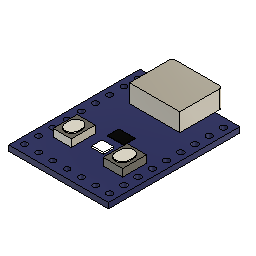
Waveshare RP2040 Zero (Autodesk Fusion 360 design; units mm, degrees)
Autodesk Fusion 360 part; units mm, degrees
sketch "Sketch1" plane through (0, 0, 0) normal (0, 0, 1) x (1, 0, 0)
  line L0 (-8.481, 10.9754) -> (9.5262, 10.9754)
  line L1 (9.5262, 10.9754) -> (9.5262, -12.7333)
  line L2 (9.5262, -12.7333) -> (-8.481, -12.7333)
  line L3 (-8.481, -12.7333) -> (-8.481, 10.9754)
  constraint horizontal L0
  constraint vertical L1
  constraint horizontal L2
  constraint vertical L3
extrude "Extrude1" add sketch "Sketch1" along normal blind 1
sketch "Sketch2" plane through (0, 0, 1) normal (0, 0, 1) x (-1, 0, 0)
  line L0 (8.481, 12.7333) -> (-9.5262, 12.7333)
  line L1 (-9.5262, 12.7333) -> (-9.5262, -10.9754)
  line L2 (-9.5262, -10.9754) -> (8.481, -10.9754)
  line L3 (8.481, -10.9754) -> (8.481, 12.7333)
  line L4 (4.0143, -12.313) -> (-5.0507, -12.313)
  line L5 (-5.0507, -12.313) -> (-5.0507, -4.6154)
  line L6 (-5.0507, -4.6154) -> (4.0143, -4.6154)
  line L7 (4.0143, -4.6154) -> (4.0143, -12.313)
  dimension "d3" = 9.065
  constraint horizontal L4
  constraint vertical L5
  constraint horizontal L6
  constraint vertical L7
  measures "d3" distance of L4.start L4.end
extrude "Extrude2" add sketch "Sketch2" along normal blind 3.27 contours L2 L4 L5 L7 | L2 L5 L6 L7
sketch "Sketch3" plane through (0, 0, 1) normal (0, 0, 1) x (-1, 0, 0)
  line L0 (4.0143, -4.6154) -> (4.0143, -10.9754)
  line L1 (4.0143, -10.9754) -> (8.481, -10.9754)
  line L2 (8.481, -10.9754) -> (8.481, 12.7333)
  line L3 (8.481, 12.7333) -> (-9.5262, 12.7333)
  line L4 (-9.5262, 12.7333) -> (-9.5262, -10.9754)
  line L5 (-9.5262, -10.9754) -> (-5.0507, -10.9754)
  line L6 (-5.0507, -10.9754) -> (-5.0507, -4.6154)
  line L7 (-5.0507, -4.6154) -> (4.0143, -4.6154)
  circle A0 centre (7.1853, -9.3478) radius 0.5131
  circle A1 centre (7.1853, -6.7791) radius 0.5131
  circle A2 centre (7.1853, -4.2103) radius 0.5131
  circle A3 centre (7.1853, -1.6416) radius 0.5131
  circle A4 centre (7.1853, 0.9272) radius 0.5131
  circle A5 centre (7.1853, 3.4959) radius 0.5131
  circle A6 centre (7.1853, 6.0647) radius 0.5131
  circle A7 centre (7.1853, 8.6334) radius 0.5131
  circle A8 centre (7.1853, 11.2022) radius 0.5131
  dimension "d8" = 0
  dimension "d9" = 20.55
extrude "Extrude3" cut sketch "Sketch3" against normal blind 1 contours A0 | A1 | A2 | A3 | A4 | A5 | A6 | A7 | A8
sketch "Sketch4" plane through (0, 12.313, 0) normal (0, 1, 0) x (-1, 0, 0)
  line L0 (-5.0507, 1) -> (4.0143, 1)
  line L1 (4.0143, 1) -> (4.0143, 4.27)
  line L2 (4.0143, 4.27) -> (-5.0507, 4.27)
  line L3 (-5.0507, 4.27) -> (-5.0507, 1)
  line L4 (-4.7493, 3.8918) -> (3.7026, 3.8918)
  line L5 (3.7026, 3.8918) -> (3.7026, 1.2313)
  line L6 (3.7026, 1.2313) -> (-4.7493, 1.2313)
  line L7 (-4.7493, 1.2313) -> (-4.7493, 3.8918)
  dimension "d12" = 8.4519
  constraint horizontal L4
  constraint vertical L5
  constraint horizontal L6
  constraint vertical L7
  measures "d12" distance of L4.start L4.end
extrude "Extrude4" cut sketch "Sketch4" against normal blind 7 contours L4 L5 L6 L7
sketch "Sketch5" plane through (0, 5.313, 0) normal (0, 1, 0) x (-1, 0, 0)
  line L0 (-4.7493, 1.2313) -> (3.7026, 1.2313)
  line L1 (3.7026, 1.2313) -> (3.7026, 3.8918)
  line L2 (3.7026, 3.8918) -> (-4.7493, 3.8918)
  line L3 (-4.7493, 3.8918) -> (-4.7493, 1.2313)
  line L4 (-4.1571, 2.6965) -> (3.1998, 2.6965)
  line L5 (3.1998, 2.6965) -> (3.1998, 2.1768)
  line L6 (3.1998, 2.1768) -> (-4.1571, 2.1768)
  line L7 (-4.1571, 2.1768) -> (-4.1571, 2.6965)
  constraint horizontal L4
  constraint vertical L5
  constraint horizontal L6
  constraint vertical L7
extrude "Extrude5" add sketch "Sketch5" along normal blind 7 contours L4 L5 L6 L7
fillet "Fillet1" radius 0.45 1 edges at (5.0507, 12.313, 2.635)
fillet "Fillet2" radius 0.7 1 edges at (-4.0143, 12.313, 2.635)
sketch "Sketch6" plane through (0, 0, 1) normal (0, 0, 1) x (-1, 0, 0)
  circle A0 centre (7.1853, -4.2103) radius 0.5131
  circle A1 centre (7.1853, 6.0647) radius 0.5131
  circle A2 centre (7.1853, 8.6334) radius 0.5131
  circle A3 centre (7.1853, -1.6416) radius 0.5131
  circle A4 centre (7.1853, -6.7791) radius 0.5131
  circle A5 centre (7.1853, 3.4959) radius 0.5131
  circle A6 centre (7.1853, 11.2022) radius 0.5131
  circle A7 centre (7.1853, 0.9272) radius 0.5131
  circle A8 centre (7.1853, -9.3478) radius 0.5131
  line L0 (4.0143, -4.6154) -> (4.0143, -10.9754)
  line L1 (4.0143, -10.9754) -> (8.481, -10.9754)
  line L2 (8.481, -10.9754) -> (8.481, 12.7333)
  line L3 (8.481, 12.7333) -> (-9.5262, 12.7333)
  line L4 (-9.5262, 12.7333) -> (-9.5262, -10.9754)
  line L5 (-9.5262, -10.9754) -> (-5.0507, -10.9754)
  line L6 (-5.0507, -10.9754) -> (-5.0507, -4.6154)
  line L7 (-5.0507, -4.6154) -> (4.0143, -4.6154)
  circle A9 centre (-8.1988, -9.3488) radius 0.5473
  circle A10 centre (-8.1988, -6.78) radius 0.5473
  circle A11 centre (-8.1988, -4.2113) radius 0.5473
  circle A12 centre (-8.1988, -1.6425) radius 0.5473
  circle A13 centre (-8.1988, 0.9262) radius 0.5473
  circle A14 centre (-8.1988, 3.495) radius 0.5473
  circle A15 centre (-8.1988, 6.0637) radius 0.5473
  circle A16 centre (-8.1988, 8.6325) radius 0.5473
  circle A17 centre (-8.1988, 11.2012) radius 0.5473
  dimension "d23" = 0
  dimension "d24" = 20.55
extrude "Extrude6" cut sketch "Sketch6" against normal blind 1 contours A9 | A10 | A11 | A12 | A13 | A14 | A15 | A16 | A17
sketch "Sketch7" plane through (0, 0, 1) normal (0, 0, 1) x (-1, 0, 0)
  circle A0 centre (-8.1988, 6.0637) radius 0.5473
  circle A1 centre (-8.1988, -4.2113) radius 0.5473
  circle A2 centre (-8.1988, -6.78) radius 0.5473
  circle A3 centre (-8.1988, 3.495) radius 0.5473
  circle A4 centre (-8.1988, 8.6325) radius 0.5473
  circle A5 centre (-8.1988, -1.6425) radius 0.5473
  circle A6 centre (-8.1988, -9.3488) radius 0.5473
  circle A7 centre (-8.1988, 0.9262) radius 0.5473
  circle A8 centre (-8.1988, 11.2012) radius 0.5473
  circle A9 centre (7.1853, -4.2103) radius 0.5131
  circle A10 centre (7.1853, 6.0647) radius 0.5131
  circle A11 centre (7.1853, 8.6334) radius 0.5131
  circle A12 centre (7.1853, -1.6416) radius 0.5131
  circle A13 centre (7.1853, -6.7791) radius 0.5131
  circle A14 centre (7.1853, 3.4959) radius 0.5131
  circle A15 centre (7.1853, 11.2022) radius 0.5131
  circle A16 centre (7.1853, 0.9272) radius 0.5131
  circle A17 centre (7.1853, -9.3478) radius 0.5131
  line L0 (4.0143, -4.6154) -> (4.0143, -10.9754)
  line L1 (4.0143, -10.9754) -> (8.481, -10.9754)
  line L2 (8.481, -10.9754) -> (8.481, 12.7333)
  line L3 (8.481, 12.7333) -> (-9.5262, 12.7333)
  line L4 (-9.5262, 12.7333) -> (-9.5262, -10.9754)
  line L5 (-9.5262, -10.9754) -> (-5.0507, -10.9754)
  line L6 (-5.0507, -10.9754) -> (-5.0507, -4.6154)
  line L7 (-5.0507, -4.6154) -> (4.0143, -4.6154)
  circle A18 centre (-5.6867, 11.2133) radius 0.5016
  circle A19 centre (-3.1117, 11.2133) radius 0.5016
  circle A20 centre (-0.5367, 11.2133) radius 0.5016
  circle A21 centre (2.0383, 11.2133) radius 0.5016
  circle A22 centre (4.6133, 11.2133) radius 0.5016
  dimension "d27" = 1.0031
  dimension "d30" = 10.3
  dimension "d31" = 0
  measures "d27" diameter of A18
extrude "Extrude7" cut sketch "Sketch7" against normal blind 1 contours A18 | A19 | A20 | A21 | A22
sketch "Sketch8" plane through (0, 0, 1) normal (0, 0, 1) x (-1, 0, 0)
  circle A0 centre (-0.5367, 11.2133) radius 0.5016
  circle A1 centre (2.0383, 11.2133) radius 0.5016
  circle A2 centre (-3.1117, 11.2133) radius 0.5016
  circle A3 centre (4.6133, 11.2133) radius 0.5016
  circle A4 centre (-5.6867, 11.2133) radius 0.5016
  circle A5 centre (-8.1988, 6.0637) radius 0.5473
  circle A6 centre (-8.1988, -4.2113) radius 0.5473
  circle A7 centre (-8.1988, -6.78) radius 0.5473
  circle A8 centre (-8.1988, 3.495) radius 0.5473
  circle A9 centre (-8.1988, 8.6325) radius 0.5473
  circle A10 centre (-8.1988, -1.6425) radius 0.5473
  circle A11 centre (-8.1988, -9.3488) radius 0.5473
  circle A12 centre (-8.1988, 0.9262) radius 0.5473
  circle A13 centre (-8.1988, 11.2012) radius 0.5473
  circle A14 centre (7.1853, -4.2103) radius 0.5131
  circle A15 centre (7.1853, 6.0647) radius 0.5131
  circle A16 centre (7.1853, 8.6334) radius 0.5131
  circle A17 centre (7.1853, -1.6416) radius 0.5131
  circle A18 centre (7.1853, -6.7791) radius 0.5131
  circle A19 centre (7.1853, 3.4959) radius 0.5131
  circle A20 centre (7.1853, 11.2022) radius 0.5131
  circle A21 centre (7.1853, 0.9272) radius 0.5131
  circle A22 centre (7.1853, -9.3478) radius 0.5131
  line L0 (4.0143, -4.6154) -> (4.0143, -10.9754)
  line L1 (4.0143, -10.9754) -> (8.481, -10.9754)
  line L2 (8.481, -10.9754) -> (8.481, 12.7333)
  line L3 (8.481, 12.7333) -> (-9.5262, 12.7333)
  line L4 (-9.5262, 12.7333) -> (-9.5262, -10.9754)
  line L5 (-9.5262, -10.9754) -> (-5.0507, -10.9754)
  line L6 (-5.0507, -10.9754) -> (-5.0507, -4.6154)
  line L7 (-5.0507, -4.6154) -> (4.0143, -4.6154)
  line L8 (2.4326, 7.493) -> (5.7199, 7.493)
  line L9 (5.7199, 7.493) -> (5.7199, 3.1598)
  line L10 (5.7199, 3.1598) -> (2.4326, 3.1598)
  line L11 (2.4326, 3.1598) -> (2.4326, 7.493)
  line L12 (-6.8316, 7.493) -> (-3.3202, 7.493)
  line L13 (-3.3202, 7.493) -> (-3.3202, 3.1748)
  line L14 (-3.3202, 3.1748) -> (-6.8316, 3.1748)
  line L15 (-6.8316, 3.1748) -> (-6.8316, 7.493)
  constraint horizontal L8
  constraint vertical L9
  constraint horizontal L10
  constraint vertical L11
  constraint horizontal L12
  constraint vertical L13
  constraint horizontal L14
  constraint vertical L15
extrude "Extrude8" add sketch "Sketch8" along normal blind 1.34 contours L8 L9 L10 L11 | L12 L13 L14 L15
sketch "Sketch9" plane through (0, 0, 1) normal (0, 0, 1) x (-1, 0, 0)
  line L0 (-6.8316, 3.1748) -> (-6.8316, 7.493)
  line L1 (-6.8316, 7.493) -> (-3.3202, 7.493)
  line L2 (-3.3202, 7.493) -> (-3.3202, 3.1748)
  line L3 (-3.3202, 3.1748) -> (-6.8316, 3.1748)
  line L4 (2.4326, 3.1598) -> (2.4326, 7.493)
  line L5 (2.4326, 7.493) -> (5.7199, 7.493)
  line L6 (5.7199, 7.493) -> (5.7199, 3.1598)
  line L7 (5.7199, 3.1598) -> (2.4326, 3.1598)
  circle A0 centre (-0.5367, 11.2133) radius 0.5016
  circle A1 centre (2.0383, 11.2133) radius 0.5016
  circle A2 centre (-3.1117, 11.2133) radius 0.5016
  circle A3 centre (4.6133, 11.2133) radius 0.5016
  circle A4 centre (-5.6867, 11.2133) radius 0.5016
  circle A5 centre (-8.1988, 6.0637) radius 0.5473
  circle A6 centre (-8.1988, -4.2113) radius 0.5473
  circle A7 centre (-8.1988, -6.78) radius 0.5473
  circle A8 centre (-8.1988, 3.495) radius 0.5473
  circle A9 centre (-8.1988, 8.6325) radius 0.5473
  circle A10 centre (-8.1988, -1.6425) radius 0.5473
  circle A11 centre (-8.1988, -9.3488) radius 0.5473
  circle A12 centre (-8.1988, 0.9262) radius 0.5473
  circle A13 centre (-8.1988, 11.2012) radius 0.5473
  circle A14 centre (7.1853, -4.2103) radius 0.5131
  circle A15 centre (7.1853, 6.0647) radius 0.5131
  circle A16 centre (7.1853, 8.6334) radius 0.5131
  circle A17 centre (7.1853, -1.6416) radius 0.5131
  circle A18 centre (7.1853, -6.7791) radius 0.5131
  circle A19 centre (7.1853, 3.4959) radius 0.5131
  circle A20 centre (7.1853, 11.2022) radius 0.5131
  circle A21 centre (7.1853, 0.9272) radius 0.5131
  circle A22 centre (7.1853, -9.3478) radius 0.5131
  line L8 (4.0143, -4.6154) -> (4.0143, -10.9754)
  line L9 (4.0143, -10.9754) -> (8.481, -10.9754)
  line L10 (8.481, -10.9754) -> (8.481, 12.7333)
  line L11 (8.481, 12.7333) -> (-9.5262, 12.7333)
  line L12 (-9.5262, 12.7333) -> (-9.5262, -10.9754)
  line L13 (-9.5262, -10.9754) -> (-5.0507, -10.9754)
  line L14 (-5.0507, -10.9754) -> (-5.0507, -4.6154)
  line L15 (-5.0507, -4.6154) -> (4.0143, -4.6154)
  line L16 (-1.9669, 2.4371) -> (0.9625, 2.4371)
  line L17 (0.9625, 2.4371) -> (0.9625, 0.3676)
  line L18 (0.9625, 0.3676) -> (-1.9669, 0.3676)
  line L19 (-1.9669, 0.3676) -> (-1.9669, 2.4371)
  constraint horizontal L16
  constraint vertical L17
  constraint horizontal L18
  constraint vertical L19
extrude "Extrude9" add sketch "Sketch9" along normal blind 0.1 contours L16 L17 L18 L19
sketch "Sketch10" plane through (0, 0, 1) normal (0, 0, 1) x (-1, 0, 0)
  line L0 (-1.9669, 0.3676) -> (-1.9669, 2.4371)
  line L1 (-1.9669, 2.4371) -> (0.9625, 2.4371)
  line L2 (0.9625, 2.4371) -> (0.9625, 0.3676)
  line L3 (0.9625, 0.3676) -> (-1.9669, 0.3676)
  line L4 (-6.8316, 3.1748) -> (-6.8316, 7.493)
  line L5 (-6.8316, 7.493) -> (-3.3202, 7.493)
  line L6 (-3.3202, 7.493) -> (-3.3202, 3.1748)
  line L7 (-3.3202, 3.1748) -> (-6.8316, 3.1748)
  line L8 (2.4326, 3.1598) -> (2.4326, 7.493)
  line L9 (2.4326, 7.493) -> (5.7199, 7.493)
  line L10 (5.7199, 7.493) -> (5.7199, 3.1598)
  line L11 (5.7199, 3.1598) -> (2.4326, 3.1598)
  circle A0 centre (-0.5367, 11.2133) radius 0.5016
  circle A1 centre (2.0383, 11.2133) radius 0.5016
  circle A2 centre (-3.1117, 11.2133) radius 0.5016
  circle A3 centre (4.6133, 11.2133) radius 0.5016
  circle A4 centre (-5.6867, 11.2133) radius 0.5016
  circle A5 centre (-8.1988, 6.0637) radius 0.5473
  circle A6 centre (-8.1988, -4.2113) radius 0.5473
  circle A7 centre (-8.1988, -6.78) radius 0.5473
  circle A8 centre (-8.1988, 3.495) radius 0.5473
  circle A9 centre (-8.1988, 8.6325) radius 0.5473
  circle A10 centre (-8.1988, -1.6425) radius 0.5473
  circle A11 centre (-8.1988, -9.3488) radius 0.5473
  circle A12 centre (-8.1988, 0.9262) radius 0.5473
  circle A13 centre (-8.1988, 11.2012) radius 0.5473
  circle A14 centre (7.1853, -4.2103) radius 0.5131
  circle A15 centre (7.1853, 6.0647) radius 0.5131
  circle A16 centre (7.1853, 8.6334) radius 0.5131
  circle A17 centre (7.1853, -1.6416) radius 0.5131
  circle A18 centre (7.1853, -6.7791) radius 0.5131
  circle A19 centre (7.1853, 3.4959) radius 0.5131
  circle A20 centre (7.1853, 11.2022) radius 0.5131
  circle A21 centre (7.1853, 0.9272) radius 0.5131
  circle A22 centre (7.1853, -9.3478) radius 0.5131
  line L12 (4.0143, -4.6154) -> (4.0143, -10.9754)
  line L13 (4.0143, -10.9754) -> (8.481, -10.9754)
  line L14 (8.481, -10.9754) -> (8.481, 12.7333)
  line L15 (8.481, 12.7333) -> (-9.5262, 12.7333)
  line L16 (-9.5262, 12.7333) -> (-9.5262, -10.9754)
  line L17 (-9.5262, -10.9754) -> (-5.0507, -10.9754)
  line L18 (-5.0507, -10.9754) -> (-5.0507, -4.6154)
  line L19 (-5.0507, -4.6154) -> (4.0143, -4.6154)
  line L20 (0.5391, 3.8067) -> (-1.5595, 3.8067)
  line L21 (-1.5595, 3.8067) -> (-1.5595, 5.6576)
  line L22 (-1.5595, 5.6576) -> (0.5391, 5.6576)
  line L23 (0.5391, 5.6576) -> (0.5391, 3.8067)
  constraint horizontal L20
  constraint vertical L21
  constraint horizontal L22
  constraint vertical L23
extrude "Extrude10" add sketch "Sketch10" along normal blind 0.3 contours L20 L21 L22 L23
sketch "Sketch11" plane through (0, 0, 2.34) normal (0, 0, 1) x (-1, 0, 0)
  line L0 (-6.8316, 3.1748) -> (-3.3202, 3.1748)
  line L1 (-3.3202, 3.1748) -> (-3.3202, 7.493)
  line L2 (-3.3202, 7.493) -> (-6.8316, 7.493)
  line L3 (-6.8316, 7.493) -> (-6.8316, 3.1748)
  line L4 (-5.0813, 6.9963) -> (-5.0539, 6.9963)
  line L5 (-3.8539, 5.7963) -> (-3.8539, 4.9373)
  line L6 (-5.0539, 3.7373) -> (-5.0813, 3.7373)
  line L7 (-6.2813, 4.9373) -> (-6.2813, 5.7963)
  arc A0 (-5.0813, 6.9963) -> (-6.2813, 5.7963) centre (-5.0813, 5.7963) ccw
  arc A1 (-3.8539, 5.7963) -> (-5.0539, 6.9963) centre (-5.0539, 5.7963) ccw
  arc A2 (-5.0539, 3.7373) -> (-3.8539, 4.9373) centre (-5.0539, 4.9373) ccw
  arc A3 (-6.2813, 4.9373) -> (-5.0813, 3.7373) centre (-5.0813, 4.9373) ccw
  dimension "d40" = 1.2
  constraint horizontal L4
  constraint vertical L5
  constraint horizontal L6
  constraint vertical L7
  constraint tangent L4 A0
  constraint tangent L7 A0
  constraint tangent L4 A1
  constraint tangent L5 A1
  constraint equal A0 A1
  constraint tangent L5 A2
  constraint tangent L6 A2
  constraint equal A0 A2
  constraint tangent L6 A3
  constraint tangent L7 A3
  constraint equal A0 A3
  measures "d40" radius of A0
extrude "Extrude11" add sketch "Sketch11" along normal blind 0.2 contours L4 L5 L6 L7 A0 A1 A2 A3
sketch "Sketch12" plane through (0, 0, 2.34) normal (0, 0, 1) x (-1, 0, 0)
  line L0 (2.4326, 3.1598) -> (5.7199, 3.1598)
  line L1 (5.7199, 3.1598) -> (5.7199, 7.493)
  line L2 (5.7199, 7.493) -> (2.4326, 7.493)
  line L3 (2.4326, 7.493) -> (2.4326, 3.1598)
  line L4 (4.1694, 6.9944) -> (3.9504, 6.9944)
  line L5 (5.2504, 5.6944) -> (5.2504, 5.1343)
  line L6 (3.9504, 3.8343) -> (4.1694, 3.8343)
  line L7 (2.8694, 5.1343) -> (2.8694, 5.6944)
  line L8 (2.8694, 5.4144) -> (3.0983, 5.4144)
  line L9 (3.0983, 5.4144) -> (3.0983, 5.349)
  line L10 (3.0983, 5.349) -> (2.8694, 5.349)
  line L11 (2.8694, 5.349) -> (2.8694, 5.4144)
  arc A0 (4.1694, 6.9944) -> (2.8694, 5.6944) centre (4.1694, 5.6944) ccw
  arc A1 (5.2504, 5.6944) -> (3.9504, 6.9944) centre (3.9504, 5.6944) ccw
  arc A2 (3.9504, 3.8343) -> (5.2504, 5.1343) centre (3.9504, 5.1343) ccw
  arc A3 (2.8694, 5.1343) -> (4.1694, 3.8343) centre (4.1694, 5.1343) ccw
  dimension "d43" = 1.3
  constraint horizontal L4
  constraint vertical L5
  constraint horizontal L6
  constraint vertical L7
  constraint horizontal L8
  constraint vertical L9
  constraint horizontal L10
  constraint vertical L11
  constraint coincident L7 L8.start
  constraint tangent L4 A0
  constraint tangent L7 A0
  constraint tangent L4 A1
  constraint tangent L5 A1
  constraint equal A0 A1
  constraint tangent L5 A2
  constraint tangent L6 A2
  constraint equal A0 A2
  constraint tangent L6 A3
  constraint tangent L7 A3
  constraint equal A0 A3
  measures "d43" radius of A0
extrude "Extrude12" add sketch "Sketch12" along normal blind 0.2 contours L5 L7 L8 L9 L10 A0 A1 A2 A3 | L7 L8 L9 L10 L11
sketch "Sketch13" plane through (0, 0, 0) normal (0, 0, -1) x (1, 0, 0)
  circle A0 centre (0.5367, 11.2133) radius 0.5016
  circle A1 centre (-2.0383, 11.2133) radius 0.5016
  circle A2 centre (3.1117, 11.2133) radius 0.5016
  circle A3 centre (-4.6133, 11.2133) radius 0.5016
  circle A4 centre (5.6867, 11.2133) radius 0.5016
  circle A5 centre (8.1988, 6.0637) radius 0.5473
  circle A6 centre (8.1988, -4.2113) radius 0.5473
  circle A7 centre (8.1988, -6.78) radius 0.5473
  circle A8 centre (8.1988, 3.495) radius 0.5473
  circle A9 centre (8.1988, 8.6325) radius 0.5473
  circle A10 centre (8.1988, -1.6425) radius 0.5473
  circle A11 centre (8.1988, -9.3488) radius 0.5473
  circle A12 centre (8.1988, 0.9262) radius 0.5473
  circle A13 centre (8.1988, 11.2012) radius 0.5473
  circle A14 centre (-7.1853, -4.2103) radius 0.5131
  circle A15 centre (-7.1853, 6.0647) radius 0.5131
  circle A16 centre (-7.1853, 8.6334) radius 0.5131
  circle A17 centre (-7.1853, -1.6416) radius 0.5131
  circle A18 centre (-7.1853, -6.7791) radius 0.5131
  circle A19 centre (-7.1853, 3.4959) radius 0.5131
  circle A20 centre (-7.1853, 11.2022) radius 0.5131
  circle A21 centre (-7.1853, 0.9272) radius 0.5131
  circle A22 centre (-7.1853, -9.3478) radius 0.5131
  line L0 (9.5262, 12.7333) -> (-8.481, 12.7333)
  line L1 (-8.481, 12.7333) -> (-8.481, -10.9754)
  line L2 (-8.481, -10.9754) -> (9.5262, -10.9754)
  line L3 (9.5262, -10.9754) -> (9.5262, 12.7333)
  line L4 (-3.5845, 3.4275) -> (3.4155, 3.4275)
  line L5 (3.4155, 3.4275) -> (3.4155, -3.5725)
  line L6 (3.4155, -3.5725) -> (-3.5845, -3.5725)
  line L7 (-3.5845, -3.5725) -> (-3.5845, 3.4275)
  dimension "d46" = 7
  dimension "d47" = 7
  constraint horizontal L4
  constraint vertical L5
  constraint horizontal L6
  constraint vertical L7
  measures "d46" distance of L4.start L4.end
  measures "d47" distance of L4.start L6.end
sketch "Sketch14" plane through (0, 0, 0) normal (0, 0, -1) x (1, 0, 0)
  circle A0 centre (0.5367, 11.2133) radius 0.5016
  circle A1 centre (-2.0383, 11.2133) radius 0.5016
  circle A2 centre (3.1117, 11.2133) radius 0.5016
  circle A3 centre (-4.6133, 11.2133) radius 0.5016
  circle A4 centre (5.6867, 11.2133) radius 0.5016
  circle A5 centre (8.1988, 6.0637) radius 0.5473
  circle A6 centre (8.1988, -4.2113) radius 0.5473
  circle A7 centre (8.1988, -6.78) radius 0.5473
  circle A8 centre (8.1988, 3.495) radius 0.5473
  circle A9 centre (8.1988, 8.6325) radius 0.5473
  circle A10 centre (8.1988, -1.6425) radius 0.5473
  circle A11 centre (8.1988, -9.3488) radius 0.5473
  circle A12 centre (8.1988, 0.9262) radius 0.5473
  circle A13 centre (8.1988, 11.2012) radius 0.5473
  circle A14 centre (-7.1853, -4.2103) radius 0.5131
  circle A15 centre (-7.1853, 6.0647) radius 0.5131
  circle A16 centre (-7.1853, 8.6334) radius 0.5131
  circle A17 centre (-7.1853, -1.6416) radius 0.5131
  circle A18 centre (-7.1853, -6.7791) radius 0.5131
  circle A19 centre (-7.1853, 3.4959) radius 0.5131
  circle A20 centre (-7.1853, 11.2022) radius 0.5131
  circle A21 centre (-7.1853, 0.9272) radius 0.5131
  circle A22 centre (-7.1853, -9.3478) radius 0.5131
  line L0 (9.5262, 12.7333) -> (-8.481, 12.7333)
  line L1 (-8.481, 12.7333) -> (-8.481, -10.9754)
  line L2 (-8.481, -10.9754) -> (9.5262, -10.9754)
  line L3 (9.5262, -10.9754) -> (9.5262, 12.7333)
  line L4 (3.4155, -3.5725) -> (-3.6202, -3.5725)
  line L5 (-3.6202, -3.5725) -> (-3.6202, 3.4095)
  line L6 (-3.6202, 3.4095) -> (3.4155, 3.4095)
  line L7 (3.4155, 3.4095) -> (3.4155, -3.5725)
  point P0 (3.4155, -3.5725)
  constraint horizontal L4
  constraint vertical L5
  constraint horizontal L6
  constraint vertical L7
  constraint coincident P0 L4.start
sketch "Sketch15" plane through (0, 0, 0) normal (0, 0, -1) x (1, 0, 0)
  circle A0 centre (0.5367, 11.2133) radius 0.5016
  circle A1 centre (-2.0383, 11.2133) radius 0.5016
  circle A2 centre (3.1117, 11.2133) radius 0.5016
  circle A3 centre (-4.6133, 11.2133) radius 0.5016
  circle A4 centre (5.6867, 11.2133) radius 0.5016
  circle A5 centre (8.1988, 6.0637) radius 0.5473
  circle A6 centre (8.1988, -4.2113) radius 0.5473
  circle A7 centre (8.1988, -6.78) radius 0.5473
  circle A8 centre (8.1988, 3.495) radius 0.5473
  circle A9 centre (8.1988, 8.6325) radius 0.5473
  circle A10 centre (8.1988, -1.6425) radius 0.5473
  circle A11 centre (8.1988, -9.3488) radius 0.5473
  circle A12 centre (8.1988, 0.9262) radius 0.5473
  circle A13 centre (8.1988, 11.2012) radius 0.5473
  circle A14 centre (-7.1853, -4.2103) radius 0.5131
  circle A15 centre (-7.1853, 6.0647) radius 0.5131
  circle A16 centre (-7.1853, 8.6334) radius 0.5131
  circle A17 centre (-7.1853, -1.6416) radius 0.5131
  circle A18 centre (-7.1853, -6.7791) radius 0.5131
  circle A19 centre (-7.1853, 3.4959) radius 0.5131
  circle A20 centre (-7.1853, 11.2022) radius 0.5131
  circle A21 centre (-7.1853, 0.9272) radius 0.5131
  circle A22 centre (-7.1853, -9.3478) radius 0.5131
  line L0 (9.5262, 12.7333) -> (-8.481, 12.7333)
  line L1 (-8.481, 12.7333) -> (-8.481, -10.9754)
  line L2 (-8.481, -10.9754) -> (9.5262, -10.9754)
  line L3 (9.5262, -10.9754) -> (9.5262, 12.7333)
extrude "Extrude13" add sketch "Sketch14" along normal blind 0.5 contours L4 L5 L6 L7
sketch "Sketch16" plane through (0, 0, 0) normal (0, 0, -1) x (1, 0, 0)
  line L0 (3.4155, 3.4095) -> (3.4155, -3.5725)
  line L1 (3.4155, -3.5725) -> (-3.6202, -3.5725)
  line L2 (-3.6202, -3.5725) -> (-3.6202, 3.4095)
  line L3 (-3.6202, 3.4095) -> (3.4155, 3.4095)
  circle A0 centre (0.5367, 11.2133) radius 0.5016
  circle A1 centre (-2.0383, 11.2133) radius 0.5016
  circle A2 centre (3.1117, 11.2133) radius 0.5016
  circle A3 centre (-4.6133, 11.2133) radius 0.5016
  circle A4 centre (5.6867, 11.2133) radius 0.5016
  circle A5 centre (8.1988, 6.0637) radius 0.5473
  circle A6 centre (8.1988, -4.2113) radius 0.5473
  circle A7 centre (8.1988, -6.78) radius 0.5473
  circle A8 centre (8.1988, 3.495) radius 0.5473
  circle A9 centre (8.1988, 8.6325) radius 0.5473
  circle A10 centre (8.1988, -1.6425) radius 0.5473
  circle A11 centre (8.1988, -9.3488) radius 0.5473
  circle A12 centre (8.1988, 0.9262) radius 0.5473
  circle A13 centre (8.1988, 11.2012) radius 0.5473
  circle A14 centre (-7.1853, -4.2103) radius 0.5131
  circle A15 centre (-7.1853, 6.0647) radius 0.5131
  circle A16 centre (-7.1853, 8.6334) radius 0.5131
  circle A17 centre (-7.1853, -1.6416) radius 0.5131
  circle A18 centre (-7.1853, -6.7791) radius 0.5131
  circle A19 centre (-7.1853, 3.4959) radius 0.5131
  circle A20 centre (-7.1853, 11.2022) radius 0.5131
  circle A21 centre (-7.1853, 0.9272) radius 0.5131
  circle A22 centre (-7.1853, -9.3478) radius 0.5131
  line L4 (9.5262, 12.7333) -> (-8.481, 12.7333)
  line L5 (-8.481, 12.7333) -> (-8.481, -10.9754)
  line L6 (-8.481, -10.9754) -> (9.5262, -10.9754)
  line L7 (9.5262, -10.9754) -> (9.5262, 12.7333)
  line L8 (-1.5786, 7.2979) -> (1.4214, 7.2979)
  line L9 (1.4214, 7.2979) -> (1.4214, 5.0979)
  line L10 (1.4214, 5.0979) -> (-1.5786, 5.0979)
  line L11 (-1.5786, 5.0979) -> (-1.5786, 7.2979)
  dimension "d50" = 3
  dimension "d51" = 2.2
  constraint horizontal L8
  constraint vertical L9
  constraint horizontal L10
  constraint vertical L11
  measures "d50" distance of L8.start L8.end
  measures "d51" distance of L8.start L10.end
sketch "Sketch17" plane through (0, 0, 0) normal (0, 0, -1) x (1, 0, 0)
  line L0 (3.4155, 3.4095) -> (3.4155, -3.5725)
  line L1 (3.4155, -3.5725) -> (-3.6202, -3.5725)
  line L2 (-3.6202, -3.5725) -> (-3.6202, 3.4095)
  line L3 (-3.6202, 3.4095) -> (3.4155, 3.4095)
  circle A0 centre (0.5367, 11.2133) radius 0.5016
  circle A1 centre (-2.0383, 11.2133) radius 0.5016
  circle A2 centre (3.1117, 11.2133) radius 0.5016
  circle A3 centre (-4.6133, 11.2133) radius 0.5016
  circle A4 centre (5.6867, 11.2133) radius 0.5016
  circle A5 centre (8.1988, 6.0637) radius 0.5473
  circle A6 centre (8.1988, -4.2113) radius 0.5473
  circle A7 centre (8.1988, -6.78) radius 0.5473
  circle A8 centre (8.1988, 3.495) radius 0.5473
  circle A9 centre (8.1988, 8.6325) radius 0.5473
  circle A10 centre (8.1988, -1.6425) radius 0.5473
  circle A11 centre (8.1988, -9.3488) radius 0.5473
  circle A12 centre (8.1988, 0.9262) radius 0.5473
  circle A13 centre (8.1988, 11.2012) radius 0.5473
  circle A14 centre (-7.1853, -4.2103) radius 0.5131
  circle A15 centre (-7.1853, 6.0647) radius 0.5131
  circle A16 centre (-7.1853, 8.6334) radius 0.5131
  circle A17 centre (-7.1853, -1.6416) radius 0.5131
  circle A18 centre (-7.1853, -6.7791) radius 0.5131
  circle A19 centre (-7.1853, 3.4959) radius 0.5131
  circle A20 centre (-7.1853, 11.2022) radius 0.5131
  circle A21 centre (-7.1853, 0.9272) radius 0.5131
  circle A22 centre (-7.1853, -9.3478) radius 0.5131
  line L4 (9.5262, 12.7333) -> (-8.481, 12.7333)
  line L5 (-8.481, 12.7333) -> (-8.481, -10.9754)
  line L6 (-8.481, -10.9754) -> (9.5262, -10.9754)
  line L7 (9.5262, -10.9754) -> (9.5262, 12.7333)
  line L8 (-1.5786, 7.2979) -> (1.4214, 7.2979)
  line L9 (1.4214, 7.2979) -> (1.4214, 5.0979)
  line L10 (1.4214, 5.0979) -> (-1.5786, 5.0979)
  line L11 (-1.5786, 5.0979) -> (-1.5786, 7.2979)
  point P0 (-1.5786, 7.2979)
  point P1 (1.4214, 5.0979)
  constraint horizontal L8
  constraint vertical L9
  constraint horizontal L10
  constraint vertical L11
  constraint coincident P1 L9.end
  constraint coincident P0 L8.start
sketch "Sketch18" plane through (0, 0, 0) normal (0, 0, -1) x (1, 0, 0)
  line L0 (3.4155, 3.4095) -> (3.4155, -3.5725)
  line L1 (3.4155, -3.5725) -> (-3.6202, -3.5725)
  line L2 (-3.6202, -3.5725) -> (-3.6202, 3.4095)
  line L3 (-3.6202, 3.4095) -> (3.4155, 3.4095)
  circle A0 centre (0.5367, 11.2133) radius 0.5016
  circle A1 centre (-2.0383, 11.2133) radius 0.5016
  circle A2 centre (3.1117, 11.2133) radius 0.5016
  circle A3 centre (-4.6133, 11.2133) radius 0.5016
  circle A4 centre (5.6867, 11.2133) radius 0.5016
  circle A5 centre (8.1988, 6.0637) radius 0.5473
  circle A6 centre (8.1988, -4.2113) radius 0.5473
  circle A7 centre (8.1988, -6.78) radius 0.5473
  circle A8 centre (8.1988, 3.495) radius 0.5473
  circle A9 centre (8.1988, 8.6325) radius 0.5473
  circle A10 centre (8.1988, -1.6425) radius 0.5473
  circle A11 centre (8.1988, -9.3488) radius 0.5473
  circle A12 centre (8.1988, 0.9262) radius 0.5473
  circle A13 centre (8.1988, 11.2012) radius 0.5473
  circle A14 centre (-7.1853, -4.2103) radius 0.5131
  circle A15 centre (-7.1853, 6.0647) radius 0.5131
  circle A16 centre (-7.1853, 8.6334) radius 0.5131
  circle A17 centre (-7.1853, -1.6416) radius 0.5131
  circle A18 centre (-7.1853, -6.7791) radius 0.5131
  circle A19 centre (-7.1853, 3.4959) radius 0.5131
  circle A20 centre (-7.1853, 11.2022) radius 0.5131
  circle A21 centre (-7.1853, 0.9272) radius 0.5131
  circle A22 centre (-7.1853, -9.3478) radius 0.5131
  line L4 (9.5262, 12.7333) -> (-8.481, 12.7333)
  line L5 (-8.481, 12.7333) -> (-8.481, -10.9754)
  line L6 (-8.481, -10.9754) -> (9.5262, -10.9754)
  line L7 (9.5262, -10.9754) -> (9.5262, 12.7333)
  line L8 (-1.5786, 7.2979) -> (1.4761, 7.2979)
  line L9 (1.4761, 7.2979) -> (1.4761, 5.0444)
  line L10 (1.4761, 5.0444) -> (-1.5786, 5.0444)
  line L11 (-1.5786, 5.0444) -> (-1.5786, 7.2979)
  point P0 (-1.5786, 7.2979)
  constraint horizontal L8
  constraint vertical L9
  constraint horizontal L10
  constraint vertical L11
  constraint coincident P0 L8.start
sketch "Sketch19" plane through (0, 0, 0) normal (0, 0, -1) x (1, 0, 0)
  line L0 (3.4155, 3.4095) -> (3.4155, -3.5725)
  line L1 (3.4155, -3.5725) -> (-3.6202, -3.5725)
  line L2 (-3.6202, -3.5725) -> (-3.6202, 3.4095)
  line L3 (-3.6202, 3.4095) -> (3.4155, 3.4095)
  circle A0 centre (0.5367, 11.2133) radius 0.5016
  circle A1 centre (-2.0383, 11.2133) radius 0.5016
  circle A2 centre (3.1117, 11.2133) radius 0.5016
  circle A3 centre (-4.6133, 11.2133) radius 0.5016
  circle A4 centre (5.6867, 11.2133) radius 0.5016
  circle A5 centre (8.1988, 6.0637) radius 0.5473
  circle A6 centre (8.1988, -4.2113) radius 0.5473
  circle A7 centre (8.1988, -6.78) radius 0.5473
  circle A8 centre (8.1988, 3.495) radius 0.5473
  circle A9 centre (8.1988, 8.6325) radius 0.5473
  circle A10 centre (8.1988, -1.6425) radius 0.5473
  circle A11 centre (8.1988, -9.3488) radius 0.5473
  circle A12 centre (8.1988, 0.9262) radius 0.5473
  circle A13 centre (8.1988, 11.2012) radius 0.5473
  circle A14 centre (-7.1853, -4.2103) radius 0.5131
  circle A15 centre (-7.1853, 6.0647) radius 0.5131
  circle A16 centre (-7.1853, 8.6334) radius 0.5131
  circle A17 centre (-7.1853, -1.6416) radius 0.5131
  circle A18 centre (-7.1853, -6.7791) radius 0.5131
  circle A19 centre (-7.1853, 3.4959) radius 0.5131
  circle A20 centre (-7.1853, 11.2022) radius 0.5131
  circle A21 centre (-7.1853, 0.9272) radius 0.5131
  circle A22 centre (-7.1853, -9.3478) radius 0.5131
  line L4 (9.5262, 12.7333) -> (-8.481, 12.7333)
  line L5 (-8.481, 12.7333) -> (-8.481, -10.9754)
  line L6 (-8.481, -10.9754) -> (9.5262, -10.9754)
  line L7 (9.5262, -10.9754) -> (9.5262, 12.7333)
  line L8 (-1.5786, 7.2979) -> (1.4031, 7.2979)
  line L9 (1.4031, 7.2979) -> (1.4031, 5.0444)
  line L10 (1.4031, 5.0444) -> (-1.5786, 5.0444)
  line L11 (-1.5786, 5.0444) -> (-1.5786, 7.2979)
  point P0 (-1.5786, 7.2979)
  constraint horizontal L8
  constraint vertical L9
  constraint horizontal L10
  constraint vertical L11
  constraint coincident P0 L8.start
sketch "Sketch20" plane through (0, 0, 0) normal (0, 0, -1) x (1, 0, 0)
  line L0 (3.4155, 3.4095) -> (3.4155, -3.5725)
  line L1 (3.4155, -3.5725) -> (-3.6202, -3.5725)
  line L2 (-3.6202, -3.5725) -> (-3.6202, 3.4095)
  line L3 (-3.6202, 3.4095) -> (3.4155, 3.4095)
  circle A0 centre (0.5367, 11.2133) radius 0.5016
  circle A1 centre (-2.0383, 11.2133) radius 0.5016
  circle A2 centre (3.1117, 11.2133) radius 0.5016
  circle A3 centre (-4.6133, 11.2133) radius 0.5016
  circle A4 centre (5.6867, 11.2133) radius 0.5016
  circle A5 centre (8.1988, 6.0637) radius 0.5473
  circle A6 centre (8.1988, -4.2113) radius 0.5473
  circle A7 centre (8.1988, -6.78) radius 0.5473
  circle A8 centre (8.1988, 3.495) radius 0.5473
  circle A9 centre (8.1988, 8.6325) radius 0.5473
  circle A10 centre (8.1988, -1.6425) radius 0.5473
  circle A11 centre (8.1988, -9.3488) radius 0.5473
  circle A12 centre (8.1988, 0.9262) radius 0.5473
  circle A13 centre (8.1988, 11.2012) radius 0.5473
  circle A14 centre (-7.1853, -4.2103) radius 0.5131
  circle A15 centre (-7.1853, 6.0647) radius 0.5131
  circle A16 centre (-7.1853, 8.6334) radius 0.5131
  circle A17 centre (-7.1853, -1.6416) radius 0.5131
  circle A18 centre (-7.1853, -6.7791) radius 0.5131
  circle A19 centre (-7.1853, 3.4959) radius 0.5131
  circle A20 centre (-7.1853, 11.2022) radius 0.5131
  circle A21 centre (-7.1853, 0.9272) radius 0.5131
  circle A22 centre (-7.1853, -9.3478) radius 0.5131
  line L4 (9.5262, 12.7333) -> (-8.481, 12.7333)
  line L5 (-8.481, 12.7333) -> (-8.481, -10.9754)
  line L6 (-8.481, -10.9754) -> (9.5262, -10.9754)
  line L7 (9.5262, -10.9754) -> (9.5262, 12.7333)
  line L8 (-3.1892, 9.9883) -> (2.9499, 9.9883)
  line L9 (2.9499, 9.9883) -> (2.9499, 8.0021)
  line L10 (2.9499, 8.0021) -> (-3.1892, 8.0021)
  line L11 (-3.1892, 8.0021) -> (-3.1892, 9.9883)
  constraint horizontal L8
  constraint vertical L9
  constraint horizontal L10
  constraint vertical L11
extrude "Extrude14" cut sketch "Sketch13" along normal blind 85
